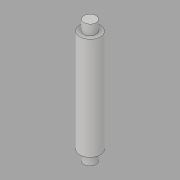
# Autodesk Inventor part: 2-2-6
Saved by Autodesk Inventor 2019 (Build 230136000, 136)
## iProperties
Created: 2020-11-06
Part Number: 2-2-6
Material: 一般
Document SubType Name: Modeling
Designer: Sugar
Density: 1 g/cm^3
Appearance: 預設
Author: Sugar
Autodesk Inventor part; units mm, degrees
ref_plane "YZ Plane" through (0, 0, 0) normal (1, 0, 0) x (0, 1, 0)
ref_plane "XZ Plane" through (0, 0, 0) normal (0, 1, 0) x (-1, 0, 0)
ref_plane "XY Plane" through (0, 0, 0) normal (0, 0, 1) x (1, 0, 0)
sketch "草圖1" plane through (0, 0, 0) normal (0, 0, 1) x (1, 0, 0)
  line L0 (-10, 50) -> (0, 50)
  line L1 (0, 50) -> (0, -50)
  line L2 (0, -50) -> (-10, -50)
  line L3 (-10, -50) -> (-10, 50)
  line L4 (-6, 60) -> (0, 60)
  line L5 (0, 60) -> (0, 50)
  line L6 (0, 50) -> (-6, 50)
  line L7 (-6, 50) -> (-6, 60)
  line L8 (-6, -50) -> (0, -50)
  line L9 (0, -50) -> (0, -60)
  line L10 (0, -60) -> (-6, -60)
  line L11 (-6, -60) -> (-6, -50)
  point P0 (0, 0)
  point P1 (0, 0)
  dimension "d1" = 10
  dimension "d2" = 120
  dimension "d3" = 100
  dimension "d4" = 6
  dimension "d5" = 6
  constraints: 24 end point, 6 parallel, 3 horizontal, 3 perpendicular, 1 coincident, 1 collinear, 1 midpoint
  measures "d1" distance between parallel lines of L1 L3
  measures "d2" distance between parallel lines of L10 L4
  measures "d3" distance of L0.end L1.end
  measures "d4" distance of L4.start L4.end
  measures "d5" distance between parallel lines of L9 L11
revolve "迴轉1" add sketch "草圖1" angle 360 about axis through (0, 50, 0) along (0, -1, 0)
